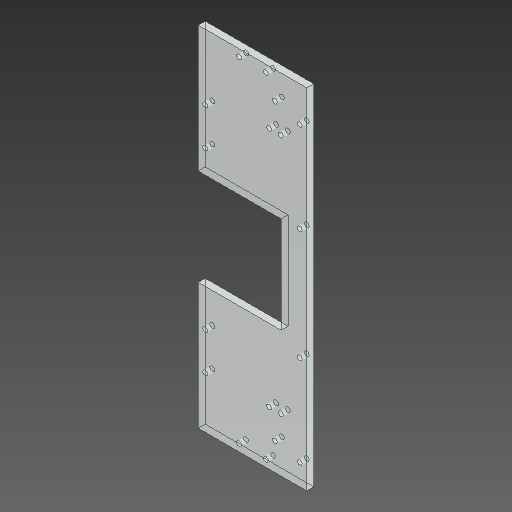
# Autodesk Inventor part: AdaptivePrintedLid
Saved by Autodesk Inventor 2021 (Build 250183000, 183)
## iProperties
Created: 2021-03-30
Part Number: AdaptivePrintedLid
Material: PBT Plastic
Document SubType Name: Modeling
Designer: Esketitttttt
Density: 1.31 g/cm^3
Appearance: Clear
Mass: 25.1744 g
Surface Area: 140.518 cm^2
Volume: 19.2171 cm^3
Author: Esketitttttt
Autodesk Inventor part; units mm, degrees
ref_plane "YZ Plane" through (0, 0, 0) normal (1, 0, 0) x (0, 1, 0)
ref_plane "XZ Plane" through (0, 0, 0) normal (0, 1, 0) x (-1, 0, 0)
ref_plane "Work Plane1" through (0, -4.7625, 0) normal (0, 0, 1) x (1, 0, 0)
sketch "Sketch1" plane through (0, -4.7625, 0) normal (0, 0, 1) x (1, 0, 0)
  circle A0 centre (-41.9763, 52.4978) radius 0.762 construction
  circle A1 centre (0.7937, 25.2604) radius 0.762 construction
  circle A2 centre (-41.9763, -52.4978) radius 0.762 construction
  circle A3 centre (0.7937, -66.2561) radius 0.762 construction
  circle A4 centre (0.7937, 66.2561) radius 0.762 construction
  circle A5 centre (0.7937, -25.2604) radius 0.762 construction
  circle A6 centre (-26.6613, 78.9561) radius 0.762 construction
  circle A7 centre (-26.6613, -72.6061) radius 0.762 construction
  circle A8 centre (-14.5213, -72.6061) radius 0.762 construction
  circle A9 centre (-14.5213, 78.9561) radius 0.762 construction
  line L0 (3.9687, -75.7811) -> (3.9687, 82.1311) projected
  line L1 (3.9687, 82.1311) -> (-45.1513, 82.1311) projected
  line L2 (-45.1513, 24.9811) -> (-45.1513, 82.1311) projected
  line L3 (-38.8013, 24.9811) -> (-45.1513, 24.9811) projected
  line L4 (-38.8013, 75.7811) -> (-38.8013, 24.9811) projected
  line L5 (-2.3813, 75.7811) -> (-38.8013, 75.7811) projected
  line L6 (-2.3813, 75.7811) -> (-2.3813, -69.4311) projected
  line L7 (-38.8013, -69.4311) -> (-2.3813, -69.4311) projected
  line L8 (-38.8013, -18.6311) -> (-38.8013, -69.4311) projected
  line L9 (-45.1513, -18.6311) -> (-38.8013, -18.6311) projected
  line L10 (-45.1513, -75.7811) -> (-45.1513, -18.6311) projected
  line L11 (3.9687, -75.7811) -> (-45.1513, -75.7811) projected
  line L12 (-3.9684, 24.9811) -> (-7.6379, 24.9811) projected
  line L13 (-3.9684, -18.6311) -> (-7.6378, -18.6311) projected
  line L14 (-38.8013, 24.9811) -> (-7.6379, 24.9811)
  line L15 (-7.6379, 24.9811) -> (-7.6378, -18.6311)
  line L16 (-7.6378, -18.6311) -> (-38.8013, -18.6311)
  circle A10 centre (-7.7531, 57.7711) radius 0.8509 projected
  circle A11 centre (-10.4351, 69.7711) radius 0.8509 projected
  circle A12 centre (-7.7531, 57.7711) radius 0.8509 projected
  circle A13 centre (-13.1131, 57.7711) radius 0.8509 projected
  circle A14 centre (-7.7531, -51.4211) radius 0.8509 projected
  circle A15 centre (-10.431, -63.4211) radius 0.8509 projected
  circle A16 centre (-13.1131, -51.4211) radius 0.8509 projected
  circle A17 centre (0.7937, 66.2561) radius 1.0922
  circle A18 centre (0.7937, 25.2604) radius 1.0922
  circle A19 centre (0.7937, -25.2604) radius 1.0922
  circle A20 centre (0.7937, -66.2561) radius 1.0922
  circle A21 centre (-14.5213, -72.6061) radius 1.0922
  circle A22 centre (-26.6613, -72.6061) radius 1.0922
  circle A23 centre (-41.9763, 52.4978) radius 1.0922
  circle A24 centre (-26.6613, 78.9561) radius 1.0922
  circle A25 centre (-14.5213, 78.9561) radius 1.0922
  circle A26 centre (-41.9763, -52.4978) radius 1.0922
  circle A27 centre (-10.4351, 69.7711) radius 1.1049
  circle A28 centre (-7.7531, 57.7711) radius 1.1049
  circle A29 centre (-13.1131, 57.7711) radius 1.1049
  circle A30 centre (-13.1131, -51.4211) radius 1.1049
  circle A31 centre (-7.7531, -51.4211) radius 1.1049
  circle A32 centre (-10.431, -63.4211) radius 1.1049
  circle A33 centre (-41.9763, 35.5644) radius 0.762 projected
  circle A34 centre (-41.9763, -35.5644) radius 0.762 projected
  circle A35 centre (-41.9763, -35.5644) radius 1.0922
  circle A36 centre (-41.9763, 35.5644) radius 1.0922
  point P0 (0, 4.7625)
  point P1 (-41.1825, -37.1519)
  point P2 (-41.1825, 37.1519)
  dimension "o" = 0.3302
  dimension "d3" = 0.3302
  dimension "d4" = 0.3302
  dimension "d5" = 0.3302
  dimension "d6" = 0.3302
  dimension "d7" = 0.3302
  dimension "d11" = 0.3302
  dimension "d12" = 0.3302
  dimension "d13" = 0.3302
  dimension "d14" = 0.3302
  dimension "d15" = 0.254
  dimension "d16" = 0.254
  dimension "d17" = 0.254
  dimension "d18" = 0.254
  dimension "d19" = 0.254
  dimension "d20" = 0.254
  dimension "d21" = 0.3302
  dimension "d22" = 0.3302
  constraints: 18 centre point, 6 end point, 1 horizontal
  measures "o" radial gap between concentric circles of A4 A17
  measures "d3" radial gap between concentric circles of A1 A18
  measures "d4" radial gap between concentric circles of A5 A19
  measures "d5" radial gap between concentric circles of A3 A20
  measures "d6" radial gap between concentric circles of A8 A21
  measures "d7" radial gap between concentric circles of A7 A22
  measures "d11" radial gap between concentric circles of A0 A23
  measures "d12" radial gap between concentric circles of A6 A24
  measures "d13" radial gap between concentric circles of A9 A25
  measures "d14" radial gap between concentric circles of A2 A26
  measures "d15" radial gap between concentric circles of A11 A27
  measures "d16" radial gap between concentric circles of A10 A28
  measures "d17" radial gap between concentric circles of A13 A29
  measures "d18" radial gap between concentric circles of A16 A30
  measures "d19" radial gap between concentric circles of A14 A31
  measures "d20" radial gap between concentric circles of A15 A32
  measures "d21" radial gap between concentric circles of A34 A35
  measures "d22" radial gap between concentric circles of A33 A36
extrude "Extrusion1" add sketch "Sketch1" along normal blind 3.175 contours L11 L10 L9 L8 L7 L6 L5 L4 L3 L2 L1 L0 | L16 L15 L14 L4 L5 L6 L7 L8
equation "\"d3\" = o"
equation "\"d4\" = o"
equation "\"d5\" = o"
equation "\"d6\" = o"
equation "\"d7\" = o"
equation "\"d11\" = o"
equation "\"d12\" = o"
equation "\"d13\" = o"
equation "\"d14\" = o"
equation "\"d21\" = o"
equation "\"d22\" = o"
body "Solid1"
